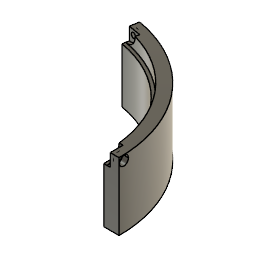
Access_Panel_1 (Autodesk Fusion 360 design; units mm, degrees)
Autodesk Fusion 360 part; units mm, degrees
sketch "Sketch1" plane through (0, 0, 0) normal (0, 0, 1) x (1, 0, 0)
  line L0 (90, 0) -> (102, 0)
  line L1 (15.6283, 88.6327) -> (17.7121, 100.4504)
  arc A0 (102, 0) -> (17.7121, 100.4504) centre (0, 0) ccw
  arc A1 (90, 0) -> (15.6283, 88.6327) centre (0, 0) ccw
  dimension "d1" = 204
  dimension "d2" = 180
  dimension "d3" = 100
  constraint coincident A0.centre A1.centre
  constraint horizontal L0
  measures "d1" diameter of A0
  measures "d2" diameter of A1
  measures "d3" angle of L0 L1
extrude "Extrude1" add sketch "Sketch1" along normal blind 43
sketch "Sketch2" plane through (0, 0, 43) normal (0, 0, 1) x (-1, 0, 0)
  arc A0 (-102, 0) -> (-17.7121, -100.4504) centre (0, 0) ccw
  line L0 (-17.7121, -100.4504) -> (-15.6283, -88.6327)
  arc A1 (-90, 0) -> (-15.6283, -88.6327) centre (0, 0) ccw
  line L1 (-90, 0) -> (-102, 0)
  line L2 (-15.6283, -88.6327) -> (-17.7121, -100.4504)
  line L3 (-90, 0) -> (-102, 0)
  arc A2 (-102, 0) -> (-17.7121, -100.4504) centre (0, 0) ccw
  arc A3 (-92.5, 0) -> (-16.0625, -91.0947) centre (0, 0) ccw
  dimension "d6" = 185
  dimension "d7" = 204
  constraint concentric A0 A3
  constraint concentric A2 A3
  constraint coincident A0.end L0.start
  constraint coincident A0.start L1.end
  constraint coincident L0 A3.end
  constraint coincident L1 A3.start
  measures "d6" diameter of A3
  measures "d7" diameter of A2
extrude "Extrude2" add sketch "Sketch2" along normal blind 10 contours A0 L0 L1 L2 L3 A2 A3
sketch "Sketch3" plane through (0, 0, 0) normal (0, -1, 0) x (1, 0, 0)
  line L0 (90, 0) -> (102, 0)
  line L1 (102, 0) -> (102, 53)
  line L2 (102, 53) -> (92.5, 53)
  line L3 (92.5, 53) -> (92.5, 43)
  line L4 (92.5, 43) -> (90, 43)
  line L5 (90, 43) -> (90, 0)
  line L6 (90, 43) -> (95, 43)
  line L7 (95, 43) -> (95, 53)
  line L8 (89.7973, 53) -> (90, 43)
  line L9 (89.7973, 53) -> (95, 53)
  dimension "d10" = 5
  constraint coincident L4.end L5.start
  constraint perpendicular L3 L6
  constraint coincident L2 L7.end
  constraint perpendicular L2 L7
  constraint perpendicular L7 L9
  measures "d10" distance of L4.end L6.end
revolve "Revolve1" cut sketch "Sketch3" angle 90 about axis through (89.7973, 0, 53) along (1, 0, 0) contours L3 L4 L6 L8 L9 | L2 L3 L6 L7 L9
sketch "Sketch4" plane through (95, 0, 0) normal (-1, 0, 0) x (0, -1, 0)
  line L0 (0, 43) -> (0, 53)
  line L1 (0, 53) -> (-10, 53)
  arc A0 (-10, 53) -> (0, 43) centre (0, 53) ccw
  line L2 (0, 53) -> (0, 49)
  line L3 (0, 49) -> (-4, 49)
  circle A1 centre (-4, 49) radius 2
  dimension "d12" = 4
  dimension "d13" = 4
  dimension "d14" = 4
  constraint coincident L0.end L1.start
  constraint perpendicular L1 L2
  constraint perpendicular L0 L3
  constraint coincident L3.end A1.centre
  measures "d12" distance of L0.end L2.end
  measures "d13" distance of L2.end L3.end
  measures "d14" diameter of A1
extrude "Extrude3" cut sketch "Sketch4" against normal blind 10 contours A1
sketch "Sketch5" plane through (0, 0, 0) normal (0, 1, 0) x (1, 0, 0)
sketch "Sketch6" plane through (95, 0, 0) normal (-1, 0, 0) x (0, -1, 0)
  circle A0 centre (-4, 49) radius 2
  line L0 (0, 43) -> (0, 53)
  line L1 (0, 53) -> (-10, 53)
  arc A1 (-10, 53) -> (0, 43) centre (0, 53) ccw
  circle A2 centre (-4, 49) radius 3.65
  dimension "d17" = 7.3
  constraint concentric A0 A2
  measures "d17" diameter of A2
extrude "Extrude4" cut sketch "Sketch6" along normal blind 4.5 from the near side of the face at (48.9307, 89.4974, 17.6667) contours A2
sketch "Sketch7" plane through (0, 0, 0) normal (-0.984808, 0.173648, 0) x (-0.173648, -0.984808, 0)
  line L0 (-102, 0) -> (-90, 0)
  line L1 (-90, 0) -> (-90, 43)
  line L2 (-90, 43) -> (-92.5, 43)
  line L3 (-92.5, 43) -> (-92.5, 53)
  line L4 (-92.5, 53) -> (-102, 53)
  line L5 (-102, 53) -> (-102, 0)
  line L6 (-90, 43) -> (-95, 43)
  line L7 (-95, 43) -> (-95, 53)
  line L8 (-95, 53) -> (-90, 53)
  line L9 (-90, 53) -> (-90, 43)
  dimension "d20" = 5
  dimension "d21" = 10
  dimension "d22" = 5
  constraint coincident L1.end L2.start
  constraint perpendicular L3 L6
  constraint perpendicular L4 L7
  constraint perpendicular L3 L8
  measures "d20" distance of L1.end L6.end
  measures "d21" distance of L6.end L7.end
  measures "d22" distance of L7.end L8.end
revolve "Revolve2" cut sketch "Sketch7" angle 90 about axis through (16.4966, 93.5567, 53) along (-0.173648, -0.984808, 0) contours L2 L3 L6 L8 L9 | L3 L4 L6 L7 L8
sketch "Sketch8" plane through (16.4966, 93.5567, 0) normal (-0.173648, -0.984808, 0) x (0.984808, -0.173648, 0)
  line L0 (0, 53) -> (0, 43)
  arc A0 (0, 43) -> (10, 53) centre (0, 53) ccw
  line L1 (10, 53) -> (0, 53)
  line L2 (0, 53) -> (4, 53)
  line L3 (4, 53) -> (4, 49)
  circle A1 centre (4, 49) radius 2
  dimension "d24" = 4
  dimension "d25" = 4
  dimension "d26" = 4
  constraint coincident L0.start A0.centre
  constraint perpendicular L0 L2
  constraint perpendicular L2 L3
  constraint coincident L3.end A1.centre
  measures "d24" distance of L0.start L2.end
  measures "d25" distance of L2.end L3.end
  measures "d26" diameter of A1
extrude "Extrude5" cut sketch "Sketch8" against normal blind 10 contours A1
sketch "Sketch9" plane through (16.4966, 93.5567, 0) normal (-0.173648, -0.984808, 0) x (0.984808, -0.173648, 0)
  circle A0 centre (4, 49) radius 2
  line L0 (0, 53) -> (0, 43)
  arc A1 (0, 43) -> (10, 53) centre (0, 53) ccw
  line L1 (10, 53) -> (0, 53)
  circle A2 centre (4, 49) radius 3.65
  dimension "d29" = 7.3
  constraint concentric A0 A2
  measures "d29" diameter of A2
extrude "Extrude6" cut sketch "Sketch9" along normal blind 4.5 from the near side of the face at (48.9307, 89.4974, 17.6667) contours A2
